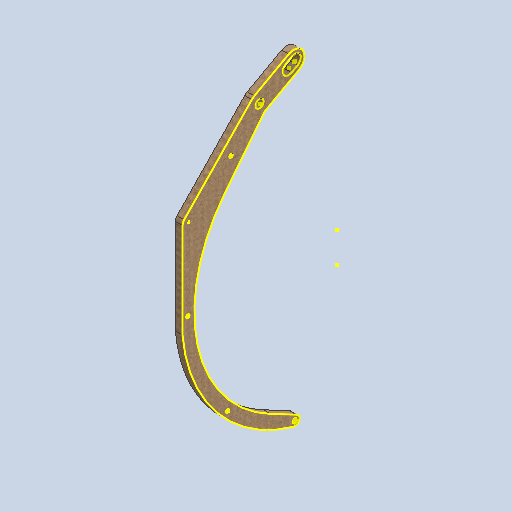
# Autodesk Inventor part: hand-grab-v1-MDF-arm
Saved by Autodesk Inventor 2025.1 (Build 291241000, 241)
## iProperties
Created: 2024-10-30
Part Number: hand-grab-v1-MDF-arm
Material: MDF 中密度繊維ボード
Document SubType Name: Modeling
Designer: haruy
Density: 0.8 g/cm^3
Appearance: ダンボール - 段ボール紙
Author: haruy
Autodesk Inventor part; units mm, degrees
ref_plane "YZ Plane" through (0, 0, 0) normal (1, 0, 0) x (0, 1, 0)
ref_plane "XZ Plane" through (0, 0, 0) normal (0, 1, 0) x (-1, 0, 0)
ref_plane "XY Plane" through (0, 0, 0) normal (0, 0, 1) x (1, 0, 0)
derived "hand-grab-v3-Sketch-Base.ipt"
sketch "スケッチ1" plane through (400, 0, 0) normal (1, 0, 0) x (0, 1, 0)
  circle A0 centre (0, 0) radius 120 construction
  circle A1 centre (-96.5237, 35.1318) radius 6.5
  line L0 (0, 0) -> (-96.5237, 35.1318)
  line L1 (0, 0) -> (0, 120)
  line L2 (246.0862, 200) -> (-251.4603, 200)
  circle A2 centre (-67.6203, 200) radius 6.5
  line L3 (0, 0) -> (-120, 0)
  line L4 (249, 9.15) -> (187, 9.15)
  line L5 (187, 9.15) -> (187, -9.15)
  line L6 (187, -9.15) -> (249, -9.15)
  line L7 (249, -9.15) -> (249, 9.15)
  line L8 (187, 5.15) -> (179, 5.15)
  line L9 (179, 5.15) -> (179, -4.85)
  line L10 (179, -4.85) -> (187, -4.85)
  line L11 (187, -4.85) -> (187, 5.15)
  line L12 (179, 3.15) -> (174, 3.15)
  line L13 (174, 3.15) -> (174, -2.85)
  line L14 (174, -2.85) -> (179, -2.85)
  line L15 (179, -2.85) -> (179, 3.15)
  line L16 (174, 2.65) -> (159, 2.65)
  line L17 (159, 2.65) -> (159, -2.35)
  line L18 (159, -2.35) -> (174, -2.35)
  line L19 (174, -2.35) -> (174, 2.65)
  line L20 (187, 34.15) -> (184, 34.15)
  line L21 (184, 34.15) -> (184, -43.5182)
  line L22 (184, -43.5182) -> (187, -43.5182)
  line L23 (187, -43.5182) -> (187, 34.15)
  circle A3 centre (150, 65) radius 4 construction
  circle A4 centre (150, 65) radius 14 construction
  line L24 (187, 34.15) -> (192, 34.15)
  line L25 (192, 34.15) -> (192, 14.15)
  line L26 (192, 14.15) -> (187, 14.15)
  line L27 (187, 14.15) -> (187, 34.15)
  line L28 (184, 34.15) -> (147.5804, 61.8148) construction
  line L29 (151.3533, 68.7641) -> (192, 54.15) construction
  line L30 (192, 54.15) -> (192, 34.15)
  line L31 (239.3868, 130) -> (-239.3868, 130)
  circle A5 centre (-96.5237, 35.1318) radius 4
  circle A6 centre (150, 65) radius 9
  line L32 (-92.7649, 33.7637) -> (-100.2825, 36.4998)
  line L33 (166, 36) -> (151, 36) construction
  circle A7 centre (151, 36) radius 5 construction
  circle A8 centre (151, 36) radius 9 construction
  circle A9 centre (-98.8174, 128.095) radius 6.5
  circle A10 centre (166, 36) radius 5 construction
  line L34 (150, 65) -> (166, 36) construction
  circle A11 centre (166, 36) radius 9
  circle A12 centre (150, 65) radius 42.121 construction
  line L35 (150, 65) -> (151, 36) construction
  line L36 (150, 65) -> (-96.5237, 35.1318) construction
  line L37 (-98.8174, 128.095) -> (150, 65) construction
  line L38 (150, 65) -> (151.4516, 22.904)
  circle A13 centre (150, 65) radius 33.121 construction
  circle A14 centre (151.1414, 31.8987) radius 9 construction
  line L39 (168.0777, 22.8987) -> (136, 22.8987)
  line L40 (175, 3.15) -> (175, -2.85)
  circle A15 centre (-96.5237, 35.1318) radius 2
  circle A16 centre (150, 65) radius 3.5
  circle A17 centre (150, 65) radius 29.0172 construction
  circle A18 centre (164.0176, 39.5932) radius 5 construction
  circle A19 centre (163.5345, 40.4687) radius 5
  line L41 (150, 65) -> (170.3477, 28.1198) construction
  circle A20 centre (166.4831, 35.1244) radius 5
  line L42 (167.9124, 42.8841) -> (170.861, 37.5398)
  line L43 (159.1566, 38.0533) -> (162.1052, 32.709)
  circle A21 centre (25, 0) radius 120
  circle A22 centre (25, 0) radius 122.5
  circle A23 centre (25, 0) radius 130.5
  line L44 (-92.7649, 33.7637) -> (-81.3303, 55.6226)
  line L45 (25, 130.5) -> (95, 130.5)
  line L46 (95, 130.5) -> (156.2451, 71.4806)
  line L47 (157.8802, 69.3477) -> (173.8802, 40.3477)
  line L48 (158.1198, 31.6523) -> (142.1198, 60.6523)
  line L49 (142.1198, 60.6523) -> (99.0503, 94.4275)
  circle A24 centre (123.9097, 89.024) radius 1.5
  circle A25 centre (25, 125.5) radius 1.5
  circle A26 centre (-61, 92) radius 1.5
  point P0 (-60, 0)
  point P1 (95.5189, 130)
  point P2 (13.5873, 130)
  point P3 (-100.3663, 36.2426)
  point P4 (-92.6811, 34.0209)
  point P5 (-92.7432, 33.8053)
  dimension "d1" = 4
  dimension "d2" = 7
  dimension "d3" = 10
  dimension "d4" = 10
  dimension "d5" = 1
  dimension "d6" = 10
  dimension "d7" = 1
  dimension "d8" = 70
  dimension "d12" = 3
  dimension "d13" = 3
  dimension "d14" = 3
  dimension "d15" = 5
  dimension "d16" = 0
  dimension "d17" = 61
  dimension "d18" = 92
  dimension "d19" = 98.9097
  dimension "d20" = 89.024
  measures "d1" diameter of A15
  measures "d2" diameter of A16
  measures "d3" diameter of A18
  measures "d4" diameter of A19
  measures "d5" distance of A19.centre A18.centre
  measures "d6" diameter of A20
  measures "d7" distance of L33.start A20.centre
  measures "d8" horizontal distance of A22.centre L45.end
  measures "d12" diameter of A24
  measures "d13" diameter of A25
  measures "d14" diameter of A26
  measures "d15" distance from line of A25.centre L45
  measures "d16" horizontal distance of A25.centre L45.start
  measures "d17" horizontal distance of A26.centre point (0, 0)
  measures "d18" distance from line of L3 A26.centre
  measures "d19" horizontal distance of A24.centre A22.centre
  measures "d20" vertical distance of A22.centre A24.centre
sketch "スケッチ2" plane through (0, 400, 0) normal (0, 1, 0) x (-1, 0, 0)
  circle A0 centre (0, 0) radius 120
  line L0 (0, 0) -> (-331.4625, 0)
  line L1 (67.5, -116.9134) -> (-135, 0)
  circle A1 centre (0, 0) radius 5
  line L2 (0, 0) -> (67.5, 116.9134)
  line L3 (0, 0) -> (67.5, -116.9134)
  line L4 (0, 0) -> (-135, 0)
  line L5 (17.0359, 37.507) -> (12.0359, 28.8468)
  line L6 (12.0359, 28.8468) -> (15.5, 26.8468)
  line L7 (15.5, 26.8468) -> (20.5, 35.507)
  line L8 (20.5, 35.507) -> (17.0359, 37.507)
  line L9 (20.5, 35.507) -> (15.5, 26.8468)
  line L10 (15.5, 26.8468) -> (18.9641, 24.8468)
  line L11 (18.9641, 24.8468) -> (23.9641, 33.507)
  line L12 (23.9641, 33.507) -> (20.5, 35.507)
  line L13 (14.5359, 33.1769) -> (21.4641, 29.1769)
  circle A2 centre (0, 0) radius 2.65
  line L14 (16.8194, 37.632) -> (10.3194, 26.3737)
  line L15 (10.3194, 26.3737) -> (5.9893, 28.8737)
  line L16 (5.9893, 28.8737) -> (12.4893, 40.132)
  line L17 (12.4893, 40.132) -> (16.8194, 37.632)
  line L18 (28.5107, 30.882) -> (24.1806, 33.382)
  line L19 (22.0107, 19.6237) -> (28.5107, 30.882)
  line L20 (24.1806, 33.382) -> (17.6806, 22.1237)
  line L21 (17.6806, 22.1237) -> (22.0107, 19.6237)
  circle A3 centre (0, 0) radius 28.3207
  line L22 (-41, 9.25) -> (-41, 4.25)
  line L23 (-41, 4.25) -> (-28, 4.25)
  line L24 (-28, 9.25) -> (-41, 9.25)
  line L25 (-28, 4.25) -> (-28, 9.25)
  line L26 (-41, -4.25) -> (-28, -4.25)
  line L27 (-41, -9.25) -> (-41, -4.25)
  line L28 (-28, -9.25) -> (-41, -9.25)
  line L29 (-28, -4.25) -> (-28, -9.25)
  line L30 (12.4893, -40.132) -> (16.8194, -37.632)
  line L31 (16.8194, -37.632) -> (10.3194, -26.3737)
  line L32 (5.9893, -28.8737) -> (12.4893, -40.132)
  line L33 (10.3194, -26.3737) -> (5.9893, -28.8737)
  line L34 (24.1806, -33.382) -> (17.6806, -22.1237)
  line L35 (28.5107, -30.882) -> (24.1806, -33.382)
  line L36 (22.0107, -19.6237) -> (28.5107, -30.882)
  line L37 (17.6806, -22.1237) -> (22.0107, -19.6237)
  line L38 (5.9893, 28.8737) -> (5.373, 27.8064)
  line L39 (22.0107, 19.6237) -> (21.3945, 18.5564)
  line L40 (-28, 9.25) -> (-26.7675, 9.25)
  line L41 (-28, -9.25) -> (-26.7675, -9.25)
  line L42 (5.9893, -28.8737) -> (2.1934, -22.2991)
  line L43 (22.0107, -19.6237) -> (21.3945, -18.5564)
  line L44 (13.6109, 31.5748) -> (3.6109, 14.2543)
  line L45 (3.6109, 14.2543) -> (-1.5853, 17.2543)
  line L46 (-1.5853, 17.2543) -> (8.4147, 34.5748)
  line L47 (8.4147, 34.5748) -> (13.6109, 31.5748)
  circle A4 centre (3.5128, 20.0844) radius 1.5
  circle A5 centre (8.5128, 28.7446) radius 1.5
  circle A6 centre (20.6372, 21.7446) radius 1.5
  circle A7 centre (15.6372, 13.0844) radius 1.5
  circle A8 centre (-29.15, 7) radius 1.5
  circle A9 centre (-19.15, 7) radius 1.5
  circle A10 centre (-19.15, -7) radius 1.5
  circle A11 centre (-29.15, -7) radius 1.5
  circle A12 centre (8.5128, -28.7446) radius 1.5
  circle A13 centre (3.5128, -20.0844) radius 1.5
  circle A14 centre (15.6372, -13.0844) radius 1.5
  circle A15 centre (20.6372, -21.7446) radius 1.5
  line L48 (1.0128, 15.7543) -> (13.6109, 31.5748)
  circle A16 centre (0, 0) radius 34.3835
  line L49 (-8, 47) -> (-188, 47)
  line L50 (-188, 47) -> (-188, 32)
  line L51 (-188, 32) -> (-8, 32)
  line L52 (-8, 32) -> (-8, 47)
ref_plane "作業平面1" through (400, 0, 0) normal (1, 0, 0) x (0, 1, 0)
ref_plane "作業平面2" through (0, 400, 0) normal (0, 1, 0) x (-1, 0, 0)
extrude "押し出し1" add sketch "スケッチ1" against normal blind 6 contours L44 A22 A1 | A1 A22 L1 A21 L44 | A22 A5 A23 A1 | A1 A23 L31 L49 A22 | A22 L49 A21 L1 | A5 L0 A15 L32 | A5 L32 A15 L0 | L31 L46 A6 L49 A23 | A6 | A6 L38 L48 | L38 A6 L47 A11 A19 L48 | A11 A19 L43 A20 L42 | A24 | A25 | A26
fillet "フィレット1" radius 5 1 edges at (397, 95.5189, 130)
extrude "押し出し2" cut sketch "スケッチ1" against normal blind 6 contours A24 | A25 | A26
sketch "スケッチ3" plane through (400, 13.5873, 130) normal (1, 0, 0) x (0, 0, -1)
  circle A0 centre (40.976, 110.3224) radius 1.5 projected
  circle A1 centre (4.5, 11.4127) radius 1.5 projected
  circle A2 centre (38, -74.5873) radius 1.5 projected
  circle A3 centre (65, 136.4127) radius 3.5 projected
  arc A4 (87.1159, 154.3251) -> (91.9467, 145.5693) centre (89.5313, 149.9472) ccw projected
  line L0 (87.1159, 154.3251) -> (92.4602, 157.2737) projected
  arc A5 (97.291, 148.5179) -> (92.4602, 157.2737) centre (94.8756, 152.8958) ccw projected
  line L1 (97.291, 148.5179) -> (91.9467, 145.5693) projected
  circle A6 centre (94.8682, -110.111) radius 2 projected
  arc A7 (1.3997, 83.384) -> (0, 79.9145) centre (5, 79.9145) ccw projected
  line L2 (0, 79.9145) -> (0, 0) projected
  arc A8 (0, 0) -> (93.7574, -113.9536) centre (130, 11.4127) ccw projected
  arc A9 (93.7574, -113.9536) -> (95.9791, -106.2683) centre (94.8682, -110.111) ccw projected
  arc A10 (95.9791, -106.2683) -> (96.1947, -106.3305) centre (130, 11.4127) ccw projected
  line L3 (96.1947, -106.3305) -> (74.3774, -94.9176) projected
  arc A11 (35.5725, 85.463) -> (74.3774, -94.9176) centre (130, 11.4127) ccw projected
  line L4 (35.5725, 85.463) -> (69.3477, 128.5325) projected
  line L5 (69.3477, 128.5325) -> (98.3477, 144.5325) projected
  arc A12 (98.3477, 144.5325) -> (89.6523, 160.2929) centre (94, 152.4127) ccw projected
  line L6 (89.6523, 160.2929) -> (60.6523, 144.2929) projected
  arc A13 (60.6523, 144.2929) -> (58.5194, 142.6578) centre (65, 136.4127) ccw projected
  line L7 (58.5194, 142.6578) -> (1.3997, 83.384) projected
  point P0 (130, -13.5873)
